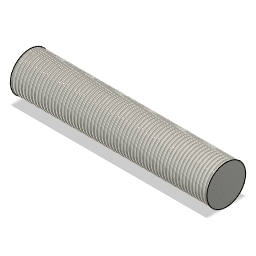
Support disipateur v1 (Autodesk Fusion 360 design; units mm, degrees)
Autodesk Fusion 360 part; units mm, degrees
sketch "Esquisse1" plane through (0, 0, 0) normal (1, 0, 0) x (0, 0, -1)
  circle A0 centre (0, 0) radius 3
  dimension "d1" = 6
  constraint coincident A0.centre origin
  measures "d1" diameter of A0
extrude "Extrusion1" add sketch "Esquisse1" along normal blind 30
thread "Filetage1" "ISO Metric profile 6.0 M6x0.5 6g" major diameter 5.927 minor diameter 5.3505 pitch 0.5 angle 60 resizes the face on face at (20, -0.2987, -2.9851)
